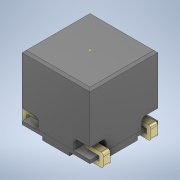
# Autodesk Inventor part: Деталь2
Saved by Autodesk Inventor 2020 (Build 240168000, 168)
## iProperties
Created: 2020-02-28
Part Number: Деталь2
Material: Типовые
Document SubType Name: Modeling
Designer: Andre
Density: 1 g/cm^3
Appearance: По умолчанию
Author: Andre
Autodesk Inventor part; units mm, degrees
ref_plane "YZ Plane" through (0, 0, 0) normal (1, 0, 0) x (0, 1, 0)
ref_plane "XZ Plane" through (0, 0, 0) normal (0, 1, 0) x (-1, 0, 0)
ref_plane "XY Plane" through (0, 0, 0) normal (0, 0, 1) x (1, 0, 0)
sketch "Эскиз1" plane through (0, 0, 0) normal (0, 1, 0) x (-1, 0, 0)
  line L0 (2.5, -2.5) -> (-2.5, -2.5)
  line L1 (-2.5, -2.5) -> (-2.5, 2.5)
  line L2 (-2.5, 2.5) -> (2.5, 2.5)
  line L3 (2.5, 2.5) -> (2.5, -2.5)
  line L4 (2.5, -2.5) -> (-2.5, 2.5) construction
  line L5 (-2.5, -2.5) -> (2.5, 2.5) construction
  point P0 (0, 0)
  dimension "d0" = 5
  dimension "d1" = 5
  constraints: 12 end point, 2 midpoint, 2 parallel, 1 horizontal, 1 perpendicular
  measures "d0" distance of L1.end L2.end
  measures "d1" distance of L0.end L1.end
extrude "Выдавливание1" add sketch "Эскиз1" along normal blind 0.5
sketch "Эскиз2" plane through (0, 0, 0) normal (0, -1, 0) x (1, 0, 0)
  line L0 (1, 2.5) -> (2.5, 2.5)
  line L1 (2.5, 2.5) -> (2.5, 1)
  line L2 (2.5, 1) -> (1, 1)
  line L3 (1, 1) -> (1, 2.5)
  line L4 (1, 2.5) -> (2.5, 1) construction
  line L5 (2.5, 2.5) -> (1, 1) construction
  line L6 (-2.5, 2.5) -> (2.5, 2.5) projected
  line L7 (2.5, 2.5) -> (2.5, -2.5) projected
  line L8 (-2.5, -2.5) -> (-2.5, 2.5) projected
  line L9 (2.5, -2.5) -> (-2.5, -2.5) projected
  line L10 (-2.5, 2.5) -> (-1, 2.5)
  line L11 (-1, 2.5) -> (-1, 1)
  line L12 (-1, 1) -> (-2.5, 1)
  line L13 (-2.5, 1) -> (-2.5, 2.5)
  line L14 (-2.5, 2.5) -> (-1, 1) construction
  line L15 (-1, 2.5) -> (-2.5, 1) construction
  line L16 (1, -1) -> (2.5, -1)
  line L17 (2.5, -1) -> (2.5, -2.5)
  line L18 (2.5, -2.5) -> (1, -2.5)
  line L19 (1, -2.5) -> (1, -1)
  line L20 (-2.5, -1) -> (-1, -1)
  line L21 (-1, -1) -> (-1, -2.5)
  line L22 (-1, -2.5) -> (-2.5, -2.5)
  line L23 (-2.5, -2.5) -> (-2.5, -1)
  point P0 (0, 0)
  point P1 (1.75, 1.75)
  point P2 (-1.75, 1.75)
  point P3 (-2.5, -1)
  point P4 (-2.5, 1)
  dimension "d4" = 1.5
  dimension "d5" = 1.5
  dimension "d6" = 1.5
  dimension "d7" = 1.5
  dimension "d8" = 1.5
  dimension "d9" = 1.5
  dimension "d10" = 1.5
  dimension "d11" = 1.5
  constraints: 40 end point, 8 parallel, 4 horizontal, 4 midpoint, 4 perpendicular
  measures "d4" distance of L1.end L2.end
  measures "d5" distance of L0.end L1.end
  measures "d6" distance of L11.end L12.end
  measures "d7" distance of L10.end L11.end
  measures "d8" distance of L17.end L19.start
  measures "d9" distance of L16.end L17.end
  measures "d10" distance of L21.end L23.start
  measures "d11" distance of L20.end L21.end
extrude "Выдавливание2" cut sketch "Эскиз2" against normal blind 0.25 contours L0 L1 L2 L3 | L11 L12 L8 L6 | L7 L9 L19 L16 | L20 L21 L9 L8
sketch "Эскиз3" plane through (0, 0.5, 0) normal (0, 1, 0) x (1, 0, 0)
  line L0 (2.5, -2.5) -> (2.5, 2.5) projected
  line L1 (-2.5, 2.5) -> (2.5, 2.5)
  line L2 (2.5, 2.5) -> (2.5, -2.5)
  line L3 (2.5, -2.5) -> (-2.5, -2.5)
  line L4 (-2.5, -2.5) -> (-2.5, 2.5)
  line L5 (-2.5, 2.5) -> (2.5, -2.5) construction
  line L6 (2.5, 2.5) -> (-2.5, -2.5) construction
  point P0 (0, 0)
  constraints: 12 end point, 2 midpoint, 2 parallel, 1 horizontal, 1 perpendicular
extrude "Выдавливание3" add sketch "Эскиз3" along normal blind 0.8 separate body
sketch "Эскиз4" plane through (0, 1.3, 0) normal (0, 1, 0) x (1, 0, 0)
  line L0 (-2.5, -2.5) -> (-1, -2.5) projected
  line L1 (-2.5, -2.5) -> (-1.3, -2.5)
  line L2 (-1.3, -2.5) -> (-1.3, -1.3)
  line L3 (-1.3, -1.3) -> (-2.5, -1.3)
  line L4 (-2.5, -1.3) -> (-2.5, -2.5)
  line L5 (-2.5, -2.5) -> (2.5, -2.5) projected
  line L6 (2.5, -2.5) -> (1.3, -2.5)
  line L7 (1.3, -2.5) -> (1.3, -1.3)
  line L8 (1.3, -1.3) -> (2.5, -1.3)
  line L9 (2.5, -1.3) -> (2.5, -2.5)
  line L10 (2.5, 2.5) -> (-2.5, 2.5) projected
  line L11 (2.5, 2.5) -> (1.3, 2.5)
  line L12 (1.3, 2.5) -> (1.3, 1.3)
  line L13 (1.3, 1.3) -> (2.5, 1.3)
  line L14 (2.5, 1.3) -> (2.5, 2.5)
  line L15 (-2.5, 2.5) -> (-1.3, 2.5)
  line L16 (-1.3, 2.5) -> (-1.3, 1.3)
  line L17 (-1.3, 1.3) -> (-2.5, 1.3)
  line L18 (-2.5, 1.3) -> (-2.5, 2.5)
  point P0 (0, 0)
  dimension "d16" = 1.2
  dimension "d17" = 1.2
  dimension "d18" = 1.2
  dimension "d19" = 1.2
  dimension "d20" = 1.2
  dimension "d21" = 1.2
  dimension "d22" = 1.2
  dimension "d23" = 1.2
  constraints: 32 end point, 8 parallel, 4 horizontal, 4 perpendicular
  measures "d16" distance of L3.end L2.end
  measures "d17" distance of L2.end L1.end
  measures "d18" distance of L7.end L8.end
  measures "d19" distance of L6.end L7.end
  measures "d20" distance of L13.end L12.end
  measures "d21" distance of L12.end L11.end
  measures "d22" distance of L16.end L17.end
  measures "d23" distance of L16.end L15.end
extrude "Выдавливание4" cut sketch "Эскиз4" against normal blind 0.8 bodies 2
sketch "Эскиз5" plane through (0, 1.3, 0) normal (0, 1, 0) x (1, 0, 0)
  line L0 (2.5, -2.5) -> (2.5, 2.5) projected
  line L1 (-2.5, -2.5) -> (2.5, -2.5)
  line L2 (2.5, -2.5) -> (2.5, 2.5)
  line L3 (2.5, 2.5) -> (-2.5, 2.5)
  line L4 (-2.5, 2.5) -> (-2.5, -2.5)
  line L5 (-2.5, -2.5) -> (2.5, 2.5) construction
  line L6 (2.5, -2.5) -> (-2.5, 2.5) construction
  point P0 (0, 0)
  constraints: 12 end point, 2 midpoint, 2 parallel, 1 horizontal, 1 perpendicular
extrude "Выдавливание5" add sketch "Эскиз5" along normal blind 3.7 bodies 2
sketch "Эскиз6" plane through (0, 5, 0) normal (0, 1, 0) x (1, 0, 0)
  point P0 (0, 0)
chamfer "Фаска1" distance 0.15 angle 45 4 edges at (0, 5, 2.5) (-2.5, 5, 0) (0, 5, -2.5) (2.5, 5, 0)
fillet "Сопряжение1" radius 0.3 7 edges at (1.3, 1.3, 1.9) (-1.3, 1.3, 1.9) (1.9, 1.3, 1.3) (1.3, 1.3, -1.9) (1.9, 1.3, -1.3) (-1.9, 1.3, -1.3) (-1.3, 1.3, -1.9)
fillet "Сопряжение2" radius 0.3 3 edges at (-1.3879, 1.2121, 1.3) (-1.3, 0.75, 1.3) (-2.05, 1.3, 1.3)
sketch "Эскиз7" plane through (0, 0.25, 0) normal (0, -1, 0) x (1, 0, 0)
  line L0 (1.5, -1.5) -> (3, -1.5)
  line L1 (3, -1.5) -> (3, -2)
  line L2 (3, -2) -> (1.5, -2)
  line L3 (1.5, -2) -> (1.5, -1.5)
  line L4 (1.5, -1.5) -> (3, -2) construction
  line L5 (3, -1.5) -> (1.5, -2) construction
  line L6 (2.5, -1) -> (2.5, -2.5) projected
  line L7 (-3, -1.5) -> (-1.5, -1.5)
  line L8 (-1.5, -1.5) -> (-1.5, -2)
  line L9 (-1.5, -2) -> (-3, -2)
  line L10 (-3, -2) -> (-3, -1.5)
  line L11 (-3, -1.5) -> (-1.5, -2) construction
  line L12 (-1.5, -1.5) -> (-3, -2) construction
  line L13 (1.5, -1.5) -> (3, -1.5)
  line L14 (3, -1.5) -> (3, -2)
  line L15 (3, -2) -> (1.5, -2)
  line L16 (1.5, -2) -> (1.5, -1.5)
  line L17 (1.5, -1.5) -> (3, -2) construction
  line L18 (3, -1.5) -> (1.5, -2) construction
  line L19 (-3, -1.5) -> (-1.5, -1.5)
  line L20 (-3, -1.5) -> (-1.5, -2) construction
  line L21 (-1.5, -1.5) -> (-3, -2) construction
  line L22 (-3, -2) -> (-3, -1.5)
  line L23 (-1.5, -2) -> (-3, -2)
  line L24 (-1.5, -1.5) -> (-1.5, -2)
  line L25 (1.5, 2) -> (3, 2)
  line L26 (3, 2) -> (3, 1.5)
  line L27 (3, 1.5) -> (1.5, 1.5)
  line L28 (1.5, 1.5) -> (1.5, 2)
  line L29 (1.5, 2) -> (3, 1.5) construction
  line L30 (3, 2) -> (1.5, 1.5) construction
  line L31 (-3, 2) -> (-1.5, 2)
  line L32 (-3, 2) -> (-1.5, 1.5) construction
  line L33 (-1.5, 2) -> (-3, 1.5) construction
  line L34 (-3, 1.5) -> (-3, 2)
  line L35 (-1.5, 1.5) -> (-3, 1.5)
  line L36 (-1.5, 2) -> (-1.5, 1.5)
  line L37 (-1, 1) -> (-2.5, 1) projected
  line L38 (-2.5, 1) -> (-2.5, 1.6917)
  line L39 (-2.5, 1) -> (-2.5, 2.5) projected
  point P0 (0, 0)
  point P1 (2.25, -1.75)
  point P2 (-2.25, -1.75)
  point P3 (2.25, -1.75)
  point P4 (-2.25, -1.75)
  point P5 (2.25, 1.75)
  point P6 (-2.25, 1.75)
  point P7 (-2.5, 2)
  point P8 (-2.5, 1.5)
  dimension "d33" = 1.5
  dimension "d34" = 0.5
  dimension "d41" = 1.5
  dimension "d42" = 0.5
  dimension "d45" = 6
  dimension "d55" = 1.5
  dimension "d56" = 0.5
  dimension "d61" = 1.5
  dimension "d62" = 0.5
  dimension "d63" = 6
  dimension "d64" = 1.5
  dimension "d65" = 0.5
  dimension "d70" = 1.5
  dimension "d71" = 0.5
  constraints: 74 end point, 12 parallel, 6 horizontal, 6 perpendicular, 1 point on line
  measures "d33" distance of L1.end L2.end
  measures "d34" distance of L0.end L1.end
  measures "d41" distance of L11.end L12.end
  measures "d42" distance of L7.end L11.end
  measures "d45" distance of L1.end L12.end
  measures "d55" distance of L15.start L16.start
  measures "d56" distance of L13.end L15.start
  measures "d61" distance of L24.end L21.end
  measures "d62" distance of L24.start L24.end
  measures "d63" distance of L15.start L21.end
  measures "d64" distance of L27.start L28.start
  measures "d65" distance of L25.end L27.start
  measures "d70" distance of L36.end L33.end
  measures "d71" distance of L36.start L36.end
extrude "Выдавливание6" add sketch "Эскиз7" along normal blind 0.32 bodies 1
sketch "Эскиз8" plane through (0, 0.25, 0) normal (0, 1, 0) x (1, 0, 0)
  line L0 (2.5, 2) -> (3, 2) projected
  line L1 (3, 1.5) -> (2.5, 1.5) projected
  line L2 (3, 2) -> (2.67, 2)
  line L3 (2.67, 2) -> (2.67, 1.5)
  line L4 (2.67, 1.5) -> (3, 1.5)
  line L5 (3, 1.5) -> (3, 2)
  line L6 (3, 2) -> (2.67, 2)
  line L7 (2.67, 2) -> (2.67, 1.5)
  line L8 (2.67, 1.5) -> (3, 1.5)
  line L9 (3, 1.5) -> (3, 2)
  line L10 (3, -1.5) -> (3, -2) projected
  line L11 (3, -1.5) -> (2.8757, -1.5)
  line L12 (2.5, -1.5) -> (3, -1.5) projected
  line L13 (3, -1.5) -> (2.67, -1.5)
  line L14 (2.67, -1.5) -> (2.67, -2)
  line L15 (2.67, -2) -> (3, -2)
  line L16 (3, -2) -> (3, -1.5)
  line L17 (3, -1.5) -> (2.67, -1.5)
  line L18 (2.67, -1.5) -> (2.67, -2)
  line L19 (2.67, -2) -> (3, -2)
  line L20 (3, -2) -> (3, -1.5)
  line L21 (3, 2) -> (2.67, 2)
  line L22 (2.67, 2) -> (2.67, 1.5)
  line L23 (2.67, 1.5) -> (3, 1.5)
  line L24 (3, 1.5) -> (3, 2)
  line L25 (3, 2) -> (2.67, 2)
  line L26 (2.67, 2) -> (2.67, 1.5)
  line L27 (2.67, 1.5) -> (3, 1.5)
  line L28 (3, 1.5) -> (3, 2)
  line L29 (-2.67, -1.5) -> (-2.67, -2)
  line L30 (-2.67, -1.5) -> (-2.7943, -1.5)
  line L31 (-3, -1.5) -> (-2.67, -1.5)
  line L32 (-2.67, -1.5) -> (-3, -1.5)
  line L33 (-3, -1.5) -> (-3, -2)
  line L34 (-3, -2) -> (-2.67, -2)
  line L35 (-2.67, -2) -> (-2.67, -1.5)
  line L36 (-2.67, -1.5) -> (-3, -1.5)
  line L37 (-3, -1.5) -> (-3, -2)
  line L38 (-3, -2) -> (-2.67, -2)
  line L39 (-2.67, -2) -> (-2.67, -1.5)
  line L40 (-3, -2) -> (-3, -1.5) projected
  line L41 (-3, -2) -> (-3, -1.86)
  line L42 (-1.67, -0.5) -> (-1.67, -1)
  line L43 (-1.67, -0.5) -> (-1.7943, -0.5)
  line L44 (-2, -0.5) -> (-1.67, -0.5)
  line L45 (-1.67, -0.5) -> (-2, -0.5)
  line L46 (-1.67, -0.5) -> (-2, -0.5)
  line L47 (-2, -1) -> (-1.67, -1)
  line L48 (-1.67, -1) -> (-1.67, -0.5)
  line L49 (-2, -1) -> (-1.67, -1)
  line L50 (-1.67, -1) -> (-1.67, -0.5)
  line L51 (-2, -0.5) -> (-2, -1)
  line L52 (-2, -0.5) -> (-2, -1)
  line L53 (-2, -1) -> (-2, -0.5)
  line L54 (-2, -1) -> (-2, -0.86)
  line L55 (-0.67, 0.5) -> (-0.67, 0)
  line L56 (-0.67, 0.5) -> (-0.7943, 0.5)
  line L57 (-1, 0.5) -> (-0.67, 0.5)
  line L58 (-0.67, 0.5) -> (-1, 0.5)
  line L59 (-0.67, 0.5) -> (-1, 0.5)
  line L60 (-1, 0) -> (-0.67, 0)
  line L61 (-0.67, 0) -> (-0.67, 0.5)
  line L62 (-1, 0) -> (-0.67, 0)
  line L63 (-0.67, 0) -> (-0.67, 0.5)
  line L64 (-1, 0.5) -> (-1, 0)
  line L65 (-1, 0.5) -> (-1, 0)
  line L66 (-1, 0) -> (-1, 0.5)
  line L67 (-1, 0) -> (-1, 0.14)
  line L68 (-1.67, -0.5) -> (-1.67, -1)
  line L69 (-1.67, -0.5) -> (-1.7943, -0.5)
  line L70 (-2, -0.5) -> (-1.67, -0.5)
  line L71 (-1.67, -0.5) -> (-2, -0.5)
  line L72 (-1.67, -0.5) -> (-2, -0.5)
  line L73 (-2, -1) -> (-1.67, -1)
  line L74 (-1.67, -1) -> (-1.67, -0.5)
  line L75 (-2, -1) -> (-1.67, -1)
  line L76 (-1.67, -1) -> (-1.67, -0.5)
  line L77 (-2, -0.5) -> (-2, -1)
  line L78 (-2, -0.5) -> (-2, -1)
  line L79 (-2, -1) -> (-2, -0.5)
  line L80 (-2, -1) -> (-2, -0.86)
  line L81 (-0.67, 0.5) -> (-0.67, 0)
  line L82 (-0.67, 0.5) -> (-0.7943, 0.5)
  line L83 (-1, 0.5) -> (-0.67, 0.5)
  line L84 (-0.67, 0.5) -> (-1, 0.5)
  line L85 (-0.67, 0.5) -> (-1, 0.5)
  line L86 (-1, 0) -> (-0.67, 0)
  line L87 (-0.67, 0) -> (-0.67, 0.5)
  line L88 (-1, 0) -> (-0.67, 0)
  line L89 (-0.67, 0) -> (-0.67, 0.5)
  line L90 (-1, 0.5) -> (-1, 0)
  line L91 (-1, 0.5) -> (-1, 0)
  line L92 (-1, 0) -> (-1, 0.5)
  line L93 (-1, 0) -> (-1, 0.14)
  line L94 (0.33, 1.5) -> (0.33, 1)
  line L95 (0.33, 1.5) -> (0.2057, 1.5)
  line L96 (0, 1.5) -> (0.33, 1.5)
  line L97 (0.33, 1.5) -> (0, 1.5)
  line L98 (0.33, 1.5) -> (0, 1.5)
  line L99 (0, 1) -> (0.33, 1)
  line L100 (0.33, 1) -> (0.33, 1.5)
  line L101 (0, 1) -> (0.33, 1)
  line L102 (0.33, 1) -> (0.33, 1.5)
  line L103 (0, 1.5) -> (0, 1)
  line L104 (0, 1.5) -> (0, 1)
  line L105 (0, 1) -> (0, 1.5)
  line L106 (0, 1) -> (0, 1.14)
  line L107 (-3, 1.5) -> (-3, 2) projected
  line L108 (-3, 1.5) -> (-3, 1.6267)
  line L109 (1.33, 2.5) -> (1.33, 2)
  line L110 (1.33, 2.5) -> (1.2057, 2.5)
  line L111 (1, 2.5) -> (1.33, 2.5)
  line L112 (1.33, 2.5) -> (1, 2.5)
  line L113 (1.33, 2.5) -> (1, 2.5)
  line L114 (1, 2) -> (1.33, 2)
  line L115 (1.33, 2) -> (1.33, 2.5)
  line L116 (1, 2) -> (1.33, 2)
  line L117 (1.33, 2) -> (1.33, 2.5)
  line L118 (1, 2.5) -> (1, 2)
  line L119 (1, 2.5) -> (1, 2)
  line L120 (1, 2) -> (1, 2.5)
  line L121 (1, 2) -> (1, 2.14)
  line L122 (-2.67, 2) -> (-2.67, 1.5)
  line L123 (-2.67, 2) -> (-2.7943, 2)
  line L124 (-3, 2) -> (-2.67, 2)
  line L125 (-2.67, 2) -> (-3, 2)
  line L126 (-2.67, 2) -> (-3, 2)
  line L127 (-3, 1.5) -> (-2.67, 1.5)
  line L128 (-2.67, 1.5) -> (-2.67, 2)
  line L129 (-3, 1.5) -> (-2.67, 1.5)
  line L130 (-2.67, 1.5) -> (-2.67, 2)
  line L131 (-3, 2) -> (-3, 1.5)
  line L132 (-3, 2) -> (-3, 1.5)
  line L133 (-3, 1.5) -> (-3, 1.64)
  line L134 (-2.67, -1.5) -> (-2.67, -2)
  line L135 (-2.67, -1.5) -> (-2.7943, -1.5)
  line L136 (-3, -1.5) -> (-2.67, -1.5)
  line L137 (-2.67, -1.5) -> (-3, -1.5)
  line L138 (-2.67, -1.5) -> (-3, -1.5)
  line L139 (-3, -2) -> (-2.67, -2)
  line L140 (-2.67, -2) -> (-2.67, -1.5)
  line L141 (-3, -2) -> (-2.67, -2)
  line L142 (-2.67, -2) -> (-2.67, -1.5)
  line L143 (-3, -1.5) -> (-3, -2)
  line L144 (-3, -1.5) -> (-3, -2)
  line L145 (-3, -2) -> (-3, -1.86)
  point P0 (0, 0)
  constraints: 280 end point, 48 parallel, 33 horizontal, 24 perpendicular, 19 point on line
extrude "Выдавливание7" add sketch "Эскиз8" along normal blind 0.35 contours L0 L5 L1 L3 | L10 L15 L14 L12 L11 | L29 L34 L33 L31 L30 | L107 L124 L123 L122 L127 bodies 1
sketch "Эскиз10" plane through (0, 0.6, 0) normal (0, 1, 0) x (1, 0, 0)
  line L0 (3, -1.5) -> (2.67, -1.5) projected
  line L1 (2.67, -2) -> (3, -2) projected
  line L2 (3, -1.5) -> (3, -2)
  line L3 (3, -2) -> (1.5, -2)
  line L4 (1.5, -2) -> (1.5, -1.5)
  line L5 (1.5, -1.5) -> (3, -1.5)
  line L6 (3, 1.5) -> (3, 2) projected
  line L7 (3, 2) -> (3, 1.5)
  line L8 (3, 1.5) -> (1.5, 1.5)
  line L9 (1.5, 1.5) -> (1.5, 2)
  line L10 (1.5, 2) -> (3, 2)
  line L11 (-3, 2) -> (-3, 1.5) projected
  line L12 (-3, 1.5) -> (-3, 2)
  line L13 (-3, 2) -> (-1.5, 2)
  line L14 (-1.5, 2) -> (-1.5, 1.5)
  line L15 (-1.5, 1.5) -> (-3, 1.5)
  line L16 (-3, -2) -> (-3, -1.5)
  line L17 (-3, -1.5) -> (-1.5, -1.5)
  line L18 (-1.5, -1.5) -> (-1.5, -2)
  line L19 (-1.5, -2) -> (-3, -2)
  point P0 (0, 0)
  dimension "d77" = 1.5
  dimension "d78" = 1.5
  dimension "d79" = 1.5
  dimension "d80" = 1.5
  constraints: 32 end point, 10 equal length, 5 perpendicular, 1 vertical
  measures "d77" distance of L1.end L3.end
  measures "d78" distance of L6.start L8.end
  measures "d79" distance of L11.start L13.end
  measures "d80" distance of L16.end L17.end
extrude "Выдавливание8" add sketch "Эскиз10" along normal blind 0.3 bodies 1
sketch "Эскиз11" plane through (0, 0.9, 0) normal (0, 1, 0) x (1, 0, 0)
  line L0 (-1.5, 1.5) -> (-1.5, 2) projected
  line L1 (-2.5, 1.5) -> (-1.5, 1.5) projected
  line L2 (-1.5, 2) -> (-1.5, 1.5)
  line L3 (-1.5, 1.5) -> (-2, 1.5)
  line L4 (-2, 1.5) -> (-2, 2)
  line L5 (-2, 2) -> (-1.5, 2)
  line L6 (-1.5, -2) -> (-1.5, -1.5) projected
  line L7 (-2.5, -2) -> (-1.5, -2) projected
  line L8 (-1.5, -1.5) -> (-1.5, -2)
  line L9 (-1.5, -2) -> (-2, -2)
  line L10 (-2, -2) -> (-2, -1.5)
  line L11 (-2, -1.5) -> (-1.5, -1.5)
  line L12 (1.5, -1.5) -> (1.5, -2) projected
  line L13 (1.5, -2) -> (1.5, -1.5)
  line L14 (1.5, -1.5) -> (2, -1.5)
  line L15 (2, -1.5) -> (2, -2)
  line L16 (2, -2) -> (1.5, -2)
  line L17 (1.5, 2) -> (1.5, 1.5) projected
  line L18 (1.5, 2) -> (1.5, 1.5)
  line L19 (1.5, 1.5) -> (2, 1.5)
  line L20 (2, 1.5) -> (2, 2)
  line L21 (2, 2) -> (1.5, 2)
  point P0 (0, 0)
  constraints: 32 end point, 10 equal length, 6 perpendicular
extrude "Выдавливание9" add sketch "Эскиз11" along normal blind 0.5 bodies 1
fillet "Сопряжение3" radius 0.2 8 edges at (3, -0.07, -1.75) (3, 0.9, -1.75) (3, 0.9, 1.75) (3, -0.07, 1.75) (-3, -0.07, 1.75) (-3, -0.07, -1.75) (-3, 0.9, 1.75) (-3, 0.9, -1.75)
fillet "Сопряжение4" radius 0.2 8 edges at (1.5, 0.6, -1.75) (2, 0.9, -1.75) (2, 0.9, 1.75) (1.5, 0.6, 1.75) (-1.5, 0.6, 1.75) (-2, 0.9, 1.75) (-2, 0.9, -1.75) (-1.5, 0.6, -1.75)
